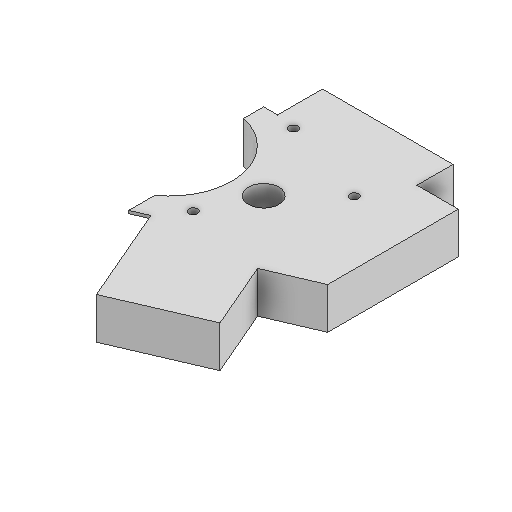
# Autodesk Inventor part: 00_KES400A_base
Saved by Autodesk Inventor 2022 (Build 260153000, 153)
## iProperties
Created: 2023-05-14
Part Number: 00_KES400A_base
Material: Generisch
Document SubType Name: Modeling
Designer: diederichbenedict
Density: 1 g/cm^3
Appearance: Vorgabe
Author: diederichbenedict
Autodesk Inventor part; units mm, degrees
ref_plane "YZ Plane" through (0, 0, 0) normal (1, 0, 0) x (0, 1, 0)
ref_plane "XZ Plane" through (0, 0, 0) normal (0, 1, 0) x (-1, 0, 0)
ref_plane "XY Plane" through (0, 0, 0) normal (0, 0, 1) x (1, 0, 0)
sketch "Skizze1" plane through (0, 0, 0) normal (0, 1, 0) x (-1, 0, 0)
  line L0 (0, 0) -> (0, -30)
  line L1 (0, -30) -> (9.5, -30)
  line L2 (9.5, -30) -> (9.5, -38.3)
  line L3 (9.5, -38.3) -> (39.5, -38.3)
  line L4 (39.5, -38.3) -> (39.5, -28)
  line L5 (39.5, -28) -> (42.7, -28)
  line L6 (42.7, -28) -> (42.7, -23.4)
  arc A0 (37.6, 2.1) -> (42.7, -23.4) centre (45.7856, -9.5229) ccw
  line L7 (0, 0) -> (11.2599, 4.8422)
  line L8 (11.2599, 4.8422) -> (4.7414, 20)
  line L9 (4.7414, 20) -> (24.5844, 28.5332)
  line L10 (24.5844, 28.5332) -> (33.3715, 8.1)
  line L11 (62.1927, -61.79) -> (-17.9865, -61.79) construction
  line L12 (-17.9865, -61.79) -> (-17.9865, 45.1157) construction
  line L13 (-17.9865, 45.1157) -> (62.1927, 45.1157) construction
  line L14 (62.1927, 45.1157) -> (62.1927, -61.79) construction
  line L15 (-1.7899, 2.1) -> (7.9361, 5.9872)
  line L16 (37.6, 2.1) -> (37.6, 8.1)
  line L17 (37.6, 8.1) -> (33.3715, 8.1)
  dimension "d0" = 30
  dimension "d1" = 9.5
  dimension "d2" = 8.3
  dimension "d3" = 30
  dimension "d4" = 10.3
  dimension "d5" = 3.2
  dimension "d6" = 4.6
  dimension "d7" = 5.1
  dimension "d8" = 25.5
  dimension "d10" = 90
  dimension "d11" = 20
  dimension "d12" = 16.5
  dimension "d13" = 21.6
  dimension "d14" = 90
  dimension "d30" = 90
  dimension "d34" = 6
  constraints: 28 end point, 6 perpendicular, 2 point on circle, 2 vertical, 1 centre point, 1 horizontal, 2 other
  measures "d0" distance of L0.start L0.end
  measures "d1" distance of L0.end L1.end
  measures "d2" distance of L1.end L2.end
  measures "d3" distance of L2.end L3.end
  measures "d4" distance of L3.end L4.end
  measures "d5" distance of L4.end L5.end
  measures "d6" distance of L5.end L6.end
  measures "d7" horizontal distance of L16.start L6.end
  measures "d8" vertical distance of L16.start L6.end
  measures "d10" angle of L7 L8
  measures "d11" vertical distance of L0.start L8.end
  measures "d12" distance from line of L7 L8.end
  measures "d13" distance of L8.end L9.end
  measures "d14" angle of L9 L10
  measures "d30" angle of L8 L9
  measures "d34" distance of L16.start L16.end
extrude "Extrusion1" add sketch "Skizze1" along normal blind 9.5
sketch "Skizze2" plane through (-24.5844, 0, 28.5332) normal (-0.9187, 0, 0.3951) x (0.3951, 0, 0.9187)
  line L0 (-22.2425, 0) -> (0, 0) projected
  line L1 (0, 0) -> (0, 9.5) projected
  line L2 (-22.2425, 9.5) -> (0, 9.5) projected
  line L3 (-22.2425, 0) -> (-22.2425, 9.5) projected
  circle A0 centre (-14.3, 4.75) radius 1.5
  point P0 (-16.5, 0)
  dimension "d38" = 14.3
  dimension "d39" = 3
  constraints: 1 centre point
  measures "d38" distance from line of A0.centre L1
  measures "d39" diameter of A0
extrude "Extrusion2" cut sketch "Skizze2" against normal blind 9.5 contours A0
sketch "Skizze3" plane through (-39.5, 0, -38.3) normal (-1, 0, 0) x (0, 0, 1)
  line L0 (0, 0) -> (10.3, 0) projected
  line L1 (10.3, 0) -> (10.3, 9.5) projected
  line L2 (0, 9.5) -> (10.3, 9.5) projected
  line L3 (0, 0) -> (0, 9.5) projected
  circle A0 centre (3, -2.3798) radius 1.5
  circle A1 centre (3, -2.3798) radius 3
  line L4 (0, 0) -> (0, 9.5) projected
  line L5 (0, -2.3798) -> (0, 0.1566)
  line L6 (6, -2.3798) -> (6, 0)
  line L7 (8.3, 0) -> (0, 0) projected
  point P0 (38.3, 0)
  dimension "d42" = 3
  dimension "d43" = 6
  constraints: 4 end point, 2 centre point, 2 point on circle, 2 point on line, 1 coincident, 1 parallel, 1 tangent
  measures "d42" diameter of A0
  measures "d43" diameter of A1
extrude "Extrusion3" add sketch "Skizze3" against normal up to surface (30 mm away) contours L6 A1 L0 | A1 L0 | A1 L5 L0 picked at (2.9397, -0.2969)
sketch "Skizze4" plane through (0, 0, 0) normal (0, -1, 0) x (1, 0, 0)
  line L0 (-39.5, -32.3) -> (-9.5, -32.3) projected
  line L1 (-9.5, -30) -> (-9.5, -32.3) projected
  line L2 (0, -30) -> (-9.5, -30) projected
  line L3 (0, 0) -> (0, -30) projected
  line L4 (-11.2599, 4.8422) -> (0, 0) projected
  line L5 (-4.7414, 20) -> (-11.2599, 4.8422) projected
  line L6 (-24.5844, 28.5332) -> (-4.7414, 20) projected
  line L7 (-33.3715, 8.1) -> (-24.5844, 28.5332) projected
  line L8 (-37.6, 8.1) -> (-33.3715, 8.1) projected
  line L9 (-37.6, 2.1) -> (-37.6, 8.1) projected
  arc A0 (-42.7, -23.4) -> (-37.6, 2.1) centre (-45.7856, -9.5229) ccw projected
  line L10 (-42.7, -28) -> (-42.7, -23.4) projected
  line L11 (-39.5, -28) -> (-42.7, -28) projected
  line L12 (-39.5, -32.3) -> (-39.5, -28) projected
  circle A1 centre (-25, -10.3) radius 3.4826
  line L13 (-39.5, -38.3) -> (-9.5, -38.3) projected
  dimension "d46" = 25
  dimension "d47" = 28
  constraints: 1 centre point
  measures "d46" distance from line of A1.centre L3
  measures "d47" distance from line of A1.centre L13
extrude "Extrusion4" cut sketch "Skizze4" against normal blind 10 contours A1
sketch "Skizze5" plane through (0, 0, 0) normal (0, -1, 0) x (1, 0, 0)
  line L0 (-9.5, -38.3) -> (-9.5, -32.3) projected
  line L1 (-39.5, -32.3) -> (-9.5, -32.3) projected
  line L2 (-39.5, -38.3) -> (-39.5, -32.3) projected
  line L3 (-39.5, -38.3) -> (-9.5, -38.3) projected
  line L4 (-9.5, -38.3) -> (-39.5, -38.3) projected
  line L5 (-35.8, -32.3) -> (-13.24, -32.3)
  line L6 (-13.24, -32.3) -> (-13.24, -38.3)
  line L7 (-13.24, -38.3) -> (-35.8, -38.3)
  line L8 (-35.8, -38.3) -> (-35.8, -32.3)
  line L9 (-13.24, -32.3) -> (-35.8, -32.3)
  line L10 (-35.8, -32.3) -> (-35.8, -38.3)
  line L11 (-35.8, -38.3) -> (-13.24, -38.3)
  line L12 (-13.24, -38.3) -> (-13.24, -32.3)
  point P0 (0, 0)
  dimension "d50" = 3.74
  dimension "d51" = 3.7
  constraints: 16 end point, 4 parallel, 2 horizontal, 2 perpendicular, 2 point on line
  measures "d50" distance between parallel lines of L6 L0
  measures "d51" distance between parallel lines of L2 L8
extrude "Extrusion5" cut sketch "Skizze5" along normal blind 10 contours L3 L8 L1 L6
sketch "Skizze6" plane through (0, 0, 0) normal (0, -1, 0) x (1, 0, 0)
  arc A0 (-36.7, -25.4555) -> (-37.7, -26.4555) centre (-36.7, -26.4555) ccw projected
  line L0 (-37.7, -26.4555) -> (-37.7, -29.6) projected
  line L1 (-37.7, -29.6) -> (-12, -29.6) projected
  line L2 (-12, -29.6) -> (-12, -20.0723) projected
  arc A1 (-12, -20.0723) -> (-13, -19.0723) centre (-13, -20.0723) ccw projected
  line L3 (-13, -19.0723) -> (-14.8624, -19.0723) projected
  arc A2 (-15.8624, -18.0723) -> (-14.8624, -19.0723) centre (-14.8624, -18.0723) ccw projected
  line L4 (-15.8624, -18.0723) -> (-15.8624, 0.4) projected
  line L5 (-15.8624, 0.4) -> (-27.397, 0.4) projected
  arc A3 (-28.397, 1.4) -> (-27.397, 0.4) centre (-27.397, 1.4) ccw projected
  line L6 (-28.397, 1.4) -> (-28.397, 2.4) projected
  arc A4 (-28.397, 2.4) -> (-29.397, 3.4) centre (-29.397, 2.4) ccw projected
  line L7 (-29.397, 3.4) -> (-31.9624, 3.4) projected
  arc A5 (-31.9624, 3.4) -> (-32.9624, 2.4) centre (-31.9624, 2.4) ccw projected
  line L8 (-32.9624, 2.4) -> (-32.9624, -24.4555) projected
  arc A6 (-33.9624, -25.4555) -> (-32.9624, -24.4555) centre (-33.9624, -24.4555) ccw projected
  line L9 (-33.9624, -25.4555) -> (-36.7, -25.4555) projected
  line L10 (-31, -17.1) -> (-31, -1.6) projected
  line L11 (-31, -1.6) -> (-17.5, -1.6) projected
  line L12 (-17.5, -1.6) -> (-17.5, -17.1) projected
  line L13 (-17.5, -17.1) -> (-31, -17.1) projected
  circle A7 centre (-35, -27.1) radius 1 projected
  circle A8 centre (-14.5, -20.6) radius 1 projected
  circle A9 centre (-30, 0.9) radius 1 projected
  line L14 (-42.7, -28) -> (-42.7, -23.4) projected
  point P0 (0, 0)
  dimension "d56" = 7.7
  measures "d56" distance from line of A7.centre L14
extrude "Extrusion6" cut sketch "Skizze6" against normal through all contours A7 | A8 | A9
sketch "Skizze7" plane through (-24.5844, 0, 28.5332) normal (-0.9187, 0, 0.3951) x (0.3951, 0, 0.9187)
  circle A0 centre (-14.3, 4.75) radius 1.5 projected
  line L0 (-22.2425, 0) -> (0, 0) projected
  line L1 (0, 0) -> (0, 9.5) projected
  line L2 (-22.2425, 9.5) -> (0, 9.5) projected
  line L3 (-22.2425, 0) -> (-22.2425, 9.5) projected
  line L4 (-29.4249, 0) -> (-23.913, 0) projected
  line L5 (-23.913, 0) -> (-23.913, 9.5) projected
  line L6 (-29.4249, 9.5) -> (-23.913, 9.5) projected
  line L7 (-29.4249, 0) -> (-29.4249, 9.5) projected
  line L8 (-23.913, 0) -> (-23.913, 9.5) projected
  line L9 (-23.913, 0) -> (-22.2425, 0) projected
  line L10 (-22.2425, 0) -> (-22.2425, 9.5) projected
  line L11 (-23.913, 9.5) -> (-22.2425, 9.5) projected
  line L12 (-23.913, 0) -> (-23.913, 9.5) projected
  line L13 (-22.2425, 0) -> (-22.2425, 9.5) projected
  line L14 (-29.4249, 0) -> (-29.4249, 9.5) projected
  line L15 (-22.2425, 1.1485) -> (-29.4249, 1.1485)
  line L16 (-29.4249, 1.1485) -> (-29.4249, 8.8348)
  line L17 (-29.4249, 8.8348) -> (-22.2425, 8.8348)
  line L18 (-22.2425, 8.8348) -> (-22.2425, 1.1485)
  point P0 (-16.5, 0)
  point P1 (-23.913, 8.8348)
  point P2 (-29.4249, 8.8348)
  point P3 (-23.913, 1.1485)
  point P4 (-23.913, 0)
  point P5 (-23.913, 9.5)
  constraints: 8 end point, 2 parallel, 2 point on line, 1 horizontal, 1 perpendicular
extrude "Extrusion7" cut sketch "Skizze7" along normal blind 10 contours L9 L5 L15 L3 | L15 L5 L17 L3 | L17 L5 L11 L3 | L15 L7 L17 L5
sketch "Skizze8" plane through (-24.5844, 0, 28.5332) normal (-0.9187, 0, 0.3951) x (0.3951, 0, 0.9187)
  line L0 (-16.5, 0) -> (-16.5, 9.5) projected
  circle A0 centre (-14.3, 4.75) radius 1.5 projected
  line L1 (0, 0) -> (-23.913, 0) projected
  line L2 (0, 0) -> (0, 9.5) projected
  line L3 (-23.913, 9.5) -> (0, 9.5) projected
  line L4 (-23.913, 9.5) -> (-23.913, 8.8348) projected
  line L5 (-23.913, 8.8348) -> (-29.4249, 8.8348) projected
  line L6 (-29.4249, 8.8348) -> (-29.4249, 1.1485) projected
  line L7 (-29.4249, 1.1485) -> (-23.913, 1.1485) projected
  line L8 (-23.913, 1.1485) -> (-23.913, 0) projected
  circle A1 centre (-24.3, 4.75) radius 1
  dimension "d59" = 2
  dimension "d60" = 10
  constraints: 1 centre point
  measures "d59" diameter of A1
  measures "d60" distance of A0.centre A1.centre
extrude "Extrusion8" cut sketch "Skizze8" against normal blind 10 contours A1
